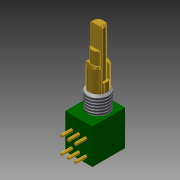
# Autodesk Inventor part: P082D
Saved by Autodesk Inventor 2016 (Build 200138000, 138)
## iProperties
Created: 2016-06-01
Part Number: P082D
Material: Generic
Document SubType Name: Modeling
Designer: Tyler
Density: 1 g/cm^3
Appearance: Gold - Metal
Author: Tyler
Autodesk Inventor part; units mm, degrees
ref_plane "YZ Plane" through (0, 0, 0) normal (1, 0, 0) x (0, 1, 0)
ref_plane "XZ Plane" through (0, 0, 0) normal (0, 1, 0) x (-1, 0, 0)
ref_plane "XY Plane" through (0, 0, 0) normal (0, 0, 1) x (1, 0, 0)
sketch "Sketch1" plane through (0, 0, 0) normal (0, 0, 1) x (1, 0, 0)
  line L0 (3.85, 3.85) -> (-3.85, 3.85)
  line L1 (-3.85, 3.85) -> (-3.85, -5.5)
  line L2 (-3.85, -5.5) -> (3.85, -5.5)
  line L3 (3.85, -5.5) -> (3.85, 3.85)
  point P0 (0, 0)
  dimension "d0" = 7.7
  dimension "d1" = 3.85
  dimension "d2" = 3.85
  dimension "d3" = 5.5
  constraints: 8 end point, 2 parallel, 1 horizontal, 1 perpendicular
  measures "d0" distance of L0.start L0.end
  measures "d1" distance from line of point (0, 0) L0
  measures "d2" distance from line of point (0, 0) L1
  measures "d3" distance from line of point (0, 0) L2
extrude "Extrusion1" add sketch "Sketch1" against normal blind 10
sketch "Sketch2" plane through (0, 0, 0) normal (0, 0, 1) x (1, 0, 0)
  circle A0 centre (0, 0) radius 3
  dimension "d6" = 6
  constraints: 1 centre point, 1 coincident
  measures "d6" diameter of A0
extrude "Extrusion2" add sketch "Sketch2" along normal blind 5
sketch "Sketch3" plane through (0, 0, 5) normal (0, 0, 1) x (1, 0, 0)
  circle A0 centre (0, 0) radius 3 projected
  circle A1 centre (0, 0) radius 2.5
  dimension "d9" = 5
  constraints: 1 centre point, 1 coincident
  measures "d9" diameter of A1
extrude "Extrusion3" add sketch "Sketch3" along normal blind 6.5 contours A1
sketch "Sketch4" plane through (0, 0, 0) normal (1, 0, 0) x (0, 1, 0)
  line L0 (1, 13.5) -> (-1, 13.5)
  line L1 (-1, 13.5) -> (-1, 7.5)
  line L2 (-1, 7.5) -> (1, 7.5)
  line L3 (1, 7.5) -> (1, 13.5)
  line L4 (2.5, 11.5) -> (-2.5, 11.5) projected
  line L5 (0, 11.5) -> (1, 13.5) construction
  line L6 (0, 11.5) -> (-1, 13.5) construction
  point P0 (0, 0)
  dimension "d12" = 2
  dimension "d13" = 4
  dimension "d14" = 2
  constraints: 12 end point, 2 parallel, 1 equal length, 1 horizontal, 1 midpoint, 1 perpendicular
  measures "d12" distance of L0.start L0.end
  measures "d13" distance between parallel lines of L4 L2
  measures "d14" distance between parallel lines of L4 L0
extrude "Extrusion4" cut sketch "Sketch4" along normal through all both and the other way through all
sketch "Sketch5" plane through (0, 0, 0) normal (0, 0, 1) x (1, 0, 0)
  circle A0 centre (0, 0) radius 3 projected
  circle A1 centre (0, 0) radius 1.75
  dimension "d17" = 3.5
  constraints: 1 centre point, 1 coincident
  measures "d17" diameter of A1
extrude "Extrusion5" add sketch "Sketch5" along normal blind 21 contours A1
sketch "Sketch6" plane through (0, 0, 21) normal (0, 0, 1) x (1, 0, 0)
  circle A0 centre (0, 0) radius 1.75 projected
  line L0 (-2, -2.75) -> (2, -2.75)
  line L1 (2, -2.75) -> (2, -0.75)
  line L2 (2, -0.75) -> (-2, -0.75)
  line L3 (-2, -0.75) -> (-2, -2.75)
  dimension "d21" = 2.5
  dimension "d22" = 2
  dimension "d23" = 2
  dimension "d24" = 2
  constraints: 8 end point, 2 parallel, 1 horizontal, 1 perpendicular
  measures "d22" distance from line of A0.centre L3
  measures "d23" distance from line of A0.centre L1
  measures "d24" distance of L0.end L1.end
extrude "Extrusion6" cut sketch "Sketch6" against normal blind 6 contours L2 A0 | A0 L2 L1 L0 L3 picked at (0.0313, -1.2733)
chamfer "Chamfer1" distance 0.5 angle 45 5 edges at (1.7073, -0.3844, 21) (-0.3844, 1.7073, 21) (0, 2.5, 11.5) (0, -2.5, 11.5) (-3, 0, 5)
sketch "Sketch7" plane through (-3.85, -5.5, 0) normal (0, -1, 0) x (1, 0, 0)
  line L0 (0, 0) -> (7.7, 0) projected
  line L1 (0, 0) -> (0, -10) projected
  line L2 (7.7, -10) -> (0, -10) projected
  line L3 (7.7, 0) -> (7.7, -10) projected
  circle A0 centre (3.85, -3.8) radius 0.4
  circle A1 centre (3.85, -8.3) radius 0.4
  circle A2 centre (5.85, -3.8) radius 0.4
  circle A3 centre (5.85, -8.3) radius 0.4
  circle A4 centre (1.85, -8.3) radius 0.4
  circle A5 centre (1.85, -3.8) radius 0.4
  line L4 (3.85, -3.8) -> (1.85, -3.8) construction
  line L5 (1.85, -8.3) -> (1.85, -3.8) construction
  line L6 (1.85, -8.3) -> (3.85, -8.3) construction
  line L7 (3.85, -8.3) -> (5.85, -8.3) construction
  line L8 (5.85, -8.3) -> (5.85, -3.8) construction
  line L9 (5.85, -3.8) -> (3.85, -3.8) construction
  point P0 (3.85, 0)
  dimension "d30" = 0.8
  dimension "d31" = 3.8
  dimension "d32" = 4.5
  dimension "d33" = 2
  dimension "d34" = 2
  dimension "d37" = 3.85
  dimension "d38" = 1.7
  constraints: 12 end point, 6 centre point, 5 equal radius, 4 perpendicular, 1 collinear, 1 parallel
  measures "d30" diameter of A0
  measures "d31" distance from line of L4.start L0
  measures "d32" distance of L6.end L4.start
  measures "d33" distance of L4.start L8.end
  measures "d34" distance of L4.start L4.end
  measures "d37" distance from line of L1 L4.start
  measures "d38" distance between parallel lines of L2 L7
extrude "Extrusion7" add sketch "Sketch7" along normal blind 3 contours A0 | A1 | A2 | A3 | A4 | A5
thread "Thread1" size "M6x0.75" class "6g" standard "ANSI Metric M Profile" full length
equation "\"d2\" = 0.5 * d0"
body "Solid1"
